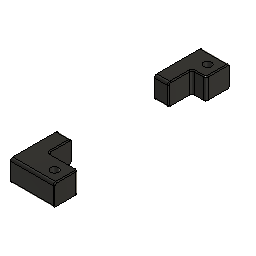
CableMount (Autodesk Fusion 360 design; units mm, degrees)
Autodesk Fusion 360 part; units mm, degrees
sketch "Sketch1" plane through (19.0523, 0, 0) normal (1, 0, 0) x (0, 1, 0)
  line L0 (120.65, 8.4918) -> (120.65, 16.9761)
  arc A0 (120.2964, 17.1226) -> (120.65, 16.9761) centre (120.65, 17.4761) ccw
  line L1 (120.2964, 17.1226) -> (118.5155, 18.9036)
  arc A1 (118.5155, 18.9036) -> (118.1619, 19.05) centre (118.1619, 18.55) ccw
  line L2 (118.1619, 19.05) -> (59.6381, 19.05)
  arc A2 (59.6381, 19.05) -> (59.2845, 18.9036) centre (59.6381, 18.55) ccw
  line L3 (59.2845, 18.9036) -> (57.5036, 17.1226)
  arc A3 (56.7964, 17.1226) -> (57.5036, 17.1226) centre (57.15, 17.4761) ccw
  line L4 (56.7964, 17.1226) -> (55.0155, 18.9036)
  arc A4 (55.0155, 18.9036) -> (54.6619, 19.05) centre (54.6619, 18.55) ccw
  line L5 (54.6619, 19.05) -> (-3.8619, 19.05)
  arc A5 (-3.8619, 19.05) -> (-4.2155, 18.9036) centre (-3.8619, 18.55) ccw
  line L6 (-4.2155, 18.9036) -> (-6.2036, 16.9155)
  arc A6 (-6.2036, 16.9155) -> (-6.35, 16.5619) centre (-5.85, 16.5619) ccw
  line L7 (-6.35, 16.5619) -> (-6.35, 7.4676)
  line L8 (-6.35, 7.4676) -> (56.1258, 7.4676)
  line L9 (56.1258, 7.4676) -> (57.15, 8.4918)
  line L10 (57.15, 8.4918) -> (58.1742, 7.4676)
  line L11 (58.1742, 7.4676) -> (119.6258, 7.4676)
  line L12 (119.6258, 7.4676) -> (120.65, 8.4918)
  line L13 (2.3114, 14.5034) -> (2.3114, 10.8966)
  arc A7 (1.8034, 10.3886) -> (2.3114, 10.8966) centre (1.8034, 10.8966) ccw
  line L14 (1.8034, 10.3886) -> (-1.8034, 10.3886)
  arc A8 (-2.3114, 10.8966) -> (-1.8034, 10.3886) centre (-1.8034, 10.8966) ccw
  line L15 (-2.3114, 10.8966) -> (-2.3114, 14.5034)
  arc A9 (-1.8034, 15.0114) -> (-2.3114, 14.5034) centre (-1.8034, 14.5034) ccw
  line L16 (-1.8034, 15.0114) -> (1.8034, 15.0114)
  arc A10 (2.3114, 14.5034) -> (1.8034, 15.0114) centre (1.8034, 14.5034) ccw
  line L17 (116.6114, 14.5034) -> (116.6114, 10.8966)
  arc A11 (116.1034, 10.3886) -> (116.6114, 10.8966) centre (116.1034, 10.8966) ccw
  line L18 (116.1034, 10.3886) -> (112.4966, 10.3886)
  arc A12 (111.9886, 10.8966) -> (112.4966, 10.3886) centre (112.4966, 10.8966) ccw
  line L19 (111.9886, 10.8966) -> (111.9886, 14.5034)
  arc A13 (112.4966, 15.0114) -> (111.9886, 14.5034) centre (112.4966, 14.5034) ccw
  line L20 (112.4966, 15.0114) -> (116.1034, 15.0114)
  arc A14 (116.6114, 14.5034) -> (116.1034, 15.0114) centre (116.1034, 14.5034) ccw
  line L21 (103.9114, 14.5034) -> (103.9114, 10.8966)
  arc A15 (103.4034, 10.3886) -> (103.9114, 10.8966) centre (103.4034, 10.8966) ccw
  line L22 (103.4034, 10.3886) -> (99.7966, 10.3886)
  arc A16 (99.2886, 10.8966) -> (99.7966, 10.3886) centre (99.7966, 10.8966) ccw
  line L23 (99.2886, 10.8966) -> (99.2886, 14.5034)
  arc A17 (99.7966, 15.0114) -> (99.2886, 14.5034) centre (99.7966, 14.5034) ccw
  line L24 (99.7966, 15.0114) -> (103.4034, 15.0114)
  arc A18 (103.9114, 14.5034) -> (103.4034, 15.0114) centre (103.4034, 14.5034) ccw
  line L25 (91.2114, 14.5034) -> (91.2114, 10.8966)
  arc A19 (90.7034, 10.3886) -> (91.2114, 10.8966) centre (90.7034, 10.8966) ccw
  line L26 (90.7034, 10.3886) -> (87.0966, 10.3886)
  arc A20 (86.5886, 10.8966) -> (87.0966, 10.3886) centre (87.0966, 10.8966) ccw
  line L27 (86.5886, 10.8966) -> (86.5886, 14.5034)
  arc A21 (87.0966, 15.0114) -> (86.5886, 14.5034) centre (87.0966, 14.5034) ccw
  line L28 (87.0966, 15.0114) -> (90.7034, 15.0114)
  arc A22 (91.2114, 14.5034) -> (90.7034, 15.0114) centre (90.7034, 14.5034) ccw
  line L29 (78.5114, 14.5034) -> (78.5114, 10.8966)
  arc A23 (78.0034, 10.3886) -> (78.5114, 10.8966) centre (78.0034, 10.8966) ccw
  line L30 (78.0034, 10.3886) -> (74.3966, 10.3886)
  arc A24 (73.8886, 10.8966) -> (74.3966, 10.3886) centre (74.3966, 10.8966) ccw
  line L31 (73.8886, 10.8966) -> (73.8886, 14.5034)
  arc A25 (74.3966, 15.0114) -> (73.8886, 14.5034) centre (74.3966, 14.5034) ccw
  line L32 (74.3966, 15.0114) -> (78.0034, 15.0114)
  arc A26 (78.5114, 14.5034) -> (78.0034, 15.0114) centre (78.0034, 14.5034) ccw
  line L33 (65.8114, 14.5034) -> (65.8114, 10.8966)
  arc A27 (65.3034, 10.3886) -> (65.8114, 10.8966) centre (65.3034, 10.8966) ccw
  line L34 (65.3034, 10.3886) -> (61.6966, 10.3886)
  arc A28 (61.1886, 10.8966) -> (61.6966, 10.3886) centre (61.6966, 10.8966) ccw
  line L35 (61.1886, 10.8966) -> (61.1886, 14.5034)
  arc A29 (61.6966, 15.0114) -> (61.1886, 14.5034) centre (61.6966, 14.5034) ccw
  line L36 (61.6966, 15.0114) -> (65.3034, 15.0114)
  arc A30 (65.8114, 14.5034) -> (65.3034, 15.0114) centre (65.3034, 14.5034) ccw
  line L37 (53.1114, 14.5034) -> (53.1114, 10.8966)
  arc A31 (52.6034, 10.3886) -> (53.1114, 10.8966) centre (52.6034, 10.8966) ccw
  line L38 (52.6034, 10.3886) -> (48.9966, 10.3886)
  arc A32 (48.4886, 10.8966) -> (48.9966, 10.3886) centre (48.9966, 10.8966) ccw
  line L39 (48.4886, 10.8966) -> (48.4886, 14.5034)
  arc A33 (48.9966, 15.0114) -> (48.4886, 14.5034) centre (48.9966, 14.5034) ccw
  line L40 (48.9966, 15.0114) -> (52.6034, 15.0114)
  arc A34 (53.1114, 14.5034) -> (52.6034, 15.0114) centre (52.6034, 14.5034) ccw
  line L41 (40.4114, 14.5034) -> (40.4114, 10.8966)
  arc A35 (39.9034, 10.3886) -> (40.4114, 10.8966) centre (39.9034, 10.8966) ccw
  line L42 (39.9034, 10.3886) -> (36.2966, 10.3886)
  arc A36 (35.7886, 10.8966) -> (36.2966, 10.3886) centre (36.2966, 10.8966) ccw
  line L43 (35.7886, 10.8966) -> (35.7886, 14.5034)
  arc A37 (36.2966, 15.0114) -> (35.7886, 14.5034) centre (36.2966, 14.5034) ccw
  line L44 (36.2966, 15.0114) -> (39.9034, 15.0114)
  arc A38 (40.4114, 14.5034) -> (39.9034, 15.0114) centre (39.9034, 14.5034) ccw
  line L45 (27.7114, 14.5034) -> (27.7114, 10.8966)
  arc A39 (27.2034, 10.3886) -> (27.7114, 10.8966) centre (27.2034, 10.8966) ccw
  line L46 (27.2034, 10.3886) -> (23.5966, 10.3886)
  arc A40 (23.0886, 10.8966) -> (23.5966, 10.3886) centre (23.5966, 10.8966) ccw
  line L47 (23.0886, 10.8966) -> (23.0886, 14.5034)
  arc A41 (23.5966, 15.0114) -> (23.0886, 14.5034) centre (23.5966, 14.5034) ccw
  line L48 (23.5966, 15.0114) -> (27.2034, 15.0114)
  arc A42 (27.7114, 14.5034) -> (27.2034, 15.0114) centre (27.2034, 14.5034) ccw
  line L49 (15.0114, 14.5034) -> (15.0114, 10.8966)
  arc A43 (14.5034, 10.3886) -> (15.0114, 10.8966) centre (14.5034, 10.8966) ccw
  line L50 (14.5034, 10.3886) -> (10.8966, 10.3886)
  arc A44 (10.3886, 10.8966) -> (10.8966, 10.3886) centre (10.8966, 10.8966) ccw
  line L51 (10.3886, 10.8966) -> (10.3886, 14.5034)
  arc A45 (10.8966, 15.0114) -> (10.3886, 14.5034) centre (10.8966, 14.5034) ccw
  line L52 (10.8966, 15.0114) -> (14.5034, 15.0114)
  arc A46 (15.0114, 14.5034) -> (14.5034, 15.0114) centre (14.5034, 14.5034) ccw
  line L53 (117.5722, 19.05) -> (119.38, 19.05)
  line L54 (120.65, 14.5095) -> (120.65, 17.78)
  line L55 (120.65, 14.5095) -> (120.65, 8.7341)
  line L56 (119.38, 7.4641) -> (96.52, 7.4641)
  line L57 (95.25, 8.7341) -> (95.25, 17.78)
  line L58 (96.52, 19.05) -> (117.5722, 19.05)
  arc A47 (120.65, 17.78) -> (119.38, 19.05) centre (119.38, 17.78) ccw
  arc A48 (119.38, 7.4641) -> (120.65, 8.7341) centre (119.38, 8.7341) ccw
  arc A49 (96.52, 19.05) -> (95.25, 17.78) centre (96.52, 17.78) ccw
  arc A50 (95.25, 8.7341) -> (96.52, 7.4641) centre (96.52, 8.7341) ccw
  point P0 (120.65, 7.4641)
  point P1 (95.25, 7.4641)
  dimension "d21" = 25.4
  dimension "d22" = 1.27
  constraint coincident L2 L53.start
  constraint coincident L0 L54.start
  constraint perpendicular L53 L54
  constraint perpendicular L11 L55
  constraint perpendicular L55 L56
  constraint perpendicular L2 L57
  constraint tangent L54 A47
  constraint tangent L53 A47
  constraint coincident P0 L55
  constraint coincident P0 L56
  constraint tangent L55 A48
  constraint tangent L56 A48
  constraint equal A47 A48
  constraint tangent L57 A49
  constraint tangent L58 A49
  constraint equal A47 A49
  constraint coincident P1 L56
  constraint coincident P1 L57
  constraint tangent L56 A50
  constraint tangent L57 A50
  constraint equal A47 A50
  measures "d21" distance of P0 P1
  measures "d22" radius of A47
extrude "Extrude1" add sketch "Sketch1" along normal blind 14.605 contours L0 A0 L1 A1 L2 L11 L12 L53 L54 L55 L57 L58 A48 A49 A50 | L12 A48 | A0 L1 A1 L53 L54 A47 | L17 A11 L18 A12 L19 A13 L20 A14 | L21 A15 L22 A16 L23 A17 L24 A18 makes body 1
sketch "Sketch2" plane through (0, 0, 7.4676) normal (0, 0, -1) x (1, 0, 0)
  line L0 (19.0523, -96.426) -> (19.0523, -119.474)
  line L1 (19.0523, -119.474) -> (33.6573, -119.474)
  line L2 (33.6573, -119.474) -> (33.6573, -96.426)
  line L3 (33.6573, -96.426) -> (19.0523, -96.426)
  line L4 (26.3548, -96.426) -> (26.3548, -107.856)
  line L5 (26.3548, -107.856) -> (33.6573, -107.856)
  line L6 (26.3548, -96.426) -> (26.3548, -95.1792)
  line L7 (26.3548, -95.1792) -> (33.6573, -95.1792)
  line L8 (33.6573, -95.1792) -> (33.6573, -107.856)
  dimension "d25" = 11.43
  dimension "d26" = 90
  constraint vertical L4
  constraint midpoint L3 L4.start
  constraint coincident L2 L5.end
  constraint perpendicular L3 L6
  constraint perpendicular L6 L7
  constraint perpendicular L5 L8
  measures "d25" distance of L4.start L4.end
  measures "d26" angle of L4 L5
extrude "Extrude2" cut sketch "Sketch2" against normal blind 29.6672 contours L3 L6 L7 L8 | L2 L3 L4 L5 L8 bodies 1
fillet "Fillet1" radius 1.27 2 edges at (26.3548, 107.856, 13.2588) (33.6573, 107.856, 13.2588) on bodies 1
fillet "Fillet2" radius 0.508 17 edges at (33.6573, 114.3, 7.4676) (33.2853, 108.228, 7.4676) (30.0061, 107.856, 7.4676) (26.7268, 107.4841, 7.4676) (26.3548, 101.506, 7.4676) (26.3548, 95.5893, 7.87) (26.3548, 95.25, 13.2571) (26.3548, 95.622, 18.678) (26.3548, 101.553, 19.05) (26.7268, 107.4841, 19.05) (30.0061, 107.856, 19.05) (33.2853, 108.228, 19.05) (33.6573, 114.253, 19.05) (33.6573, 120.278, 18.678) (33.6573, 120.65, 16.1448) (33.6573, 120.65, 11.6218) (33.6573, 120.3107, 7.87) on bodies 1
sketch "Sketch3" plane through (0, 0, 7.4676) normal (0, 0, -1) x (1, 0, 0)
  line L0 (33.1493, -119.474) -> (33.1493, -109.126)
  arc A0 (33.1493, -109.126) -> (32.3873, -108.364) centre (32.3873, -109.126) ccw
  line L1 (32.3873, -108.364) -> (27.6248, -108.364)
  arc A1 (25.8468, -106.586) -> (27.6248, -108.364) centre (27.6248, -106.586) ccw
  line L2 (25.8468, -106.586) -> (25.8468, -96.426)
  line L3 (25.8468, -96.426) -> (19.0523, -96.426)
  line L4 (19.0523, -96.426) -> (19.0523, -119.474)
  line L5 (19.0523, -119.474) -> (33.1493, -119.474)
  line L6 (30.2287, -114.3) -> (26.0385, -114.3)
  circle A2 centre (28.1336, -114.3) radius 2.0955
  dimension "d33" = 4.191
  constraint horizontal L6
  constraint midpoint L6 A2.centre
  measures "d33" diameter of A2
extrude "Extrude3" cut sketch "Sketch3" against normal blind 13.1318 contours L6 A2 | L6 A2 bodies 1
hole "Hole1" at (19.0523, 101.6, 12.7) direction (1, 0, 0) diameter 3.429 depth 6.35 tip angle 180 bodies 1
thread "Thread1" "ANSI Unified Screw Threads 0.164(#8) 8-32 UNC 8-32 UNC 2B" major diameter 4.1656 minor diameter 3.4163 pitch 0.7937 angle 60 modelled right hand crest width 0.2341 on face at (21.169, 101.738, 14.4089) crest through (19.2508, 99.8918, 12.7) on bodies 1
hole "Hole2" at (19.0523, 114.3, 12.7) direction (1, 0, 0) diameter 3.429 depth 6.35 tip angle 180 bodies 1
thread "Thread2" "ANSI Unified Screw Threads 0.164(#8) 8-32 UNC 8-32 UNC 2B" major diameter 4.1656 minor diameter 3.4163 pitch 0.7937 angle 60 modelled right hand crest width 0.2341 on face at (21.169, 115.194, 11.237) crest through (19.2508, 112.5918, 12.7) on bodies 1
sketch "Sketch4" plane through (19.0523, 0, 0) normal (1, 0, 0) x (0, 1, 0)
  line L0 (120.65, 8.4918) -> (120.65, 16.9761)
  arc A0 (120.2964, 17.1226) -> (120.65, 16.9761) centre (120.65, 17.4761) ccw
  line L1 (120.2964, 17.1226) -> (118.5155, 18.9036)
  arc A1 (118.5155, 18.9036) -> (118.1619, 19.05) centre (118.1619, 18.55) ccw
  line L2 (118.1619, 19.05) -> (59.6381, 19.05)
  arc A2 (59.6381, 19.05) -> (59.2845, 18.9036) centre (59.6381, 18.55) ccw
  line L3 (59.2845, 18.9036) -> (57.5036, 17.1226)
  arc A3 (56.7964, 17.1226) -> (57.5036, 17.1226) centre (57.15, 17.4761) ccw
  line L4 (56.7964, 17.1226) -> (55.0155, 18.9036)
  arc A4 (55.0155, 18.9036) -> (54.6619, 19.05) centre (54.6619, 18.55) ccw
  line L5 (54.6619, 19.05) -> (-3.8619, 19.05)
  arc A5 (-3.8619, 19.05) -> (-4.2155, 18.9036) centre (-3.8619, 18.55) ccw
  line L6 (-4.2155, 18.9036) -> (-6.2036, 16.9155)
  arc A6 (-6.2036, 16.9155) -> (-6.35, 16.5619) centre (-5.85, 16.5619) ccw
  line L7 (-6.35, 16.5619) -> (-6.35, 7.4676)
  line L8 (-6.35, 7.4676) -> (56.1258, 7.4676)
  line L9 (56.1258, 7.4676) -> (57.15, 8.4918)
  line L10 (57.15, 8.4918) -> (58.1742, 7.4676)
  line L11 (58.1742, 7.4676) -> (119.6258, 7.4676)
  line L12 (119.6258, 7.4676) -> (120.65, 8.4918)
  line L13 (2.3114, 14.5034) -> (2.3114, 10.8966)
  arc A7 (1.8034, 10.3886) -> (2.3114, 10.8966) centre (1.8034, 10.8966) ccw
  line L14 (1.8034, 10.3886) -> (-1.8034, 10.3886)
  arc A8 (-2.3114, 10.8966) -> (-1.8034, 10.3886) centre (-1.8034, 10.8966) ccw
  line L15 (-2.3114, 10.8966) -> (-2.3114, 14.5034)
  arc A9 (-1.8034, 15.0114) -> (-2.3114, 14.5034) centre (-1.8034, 14.5034) ccw
  line L16 (-1.8034, 15.0114) -> (1.8034, 15.0114)
  arc A10 (2.3114, 14.5034) -> (1.8034, 15.0114) centre (1.8034, 14.5034) ccw
  line L17 (116.6114, 14.5034) -> (116.6114, 10.8966)
  arc A11 (116.1034, 10.3886) -> (116.6114, 10.8966) centre (116.1034, 10.8966) ccw
  line L18 (116.1034, 10.3886) -> (112.4966, 10.3886)
  arc A12 (111.9886, 10.8966) -> (112.4966, 10.3886) centre (112.4966, 10.8966) ccw
  line L19 (111.9886, 10.8966) -> (111.9886, 14.5034)
  arc A13 (112.4966, 15.0114) -> (111.9886, 14.5034) centre (112.4966, 14.5034) ccw
  line L20 (112.4966, 15.0114) -> (116.1034, 15.0114)
  arc A14 (116.6114, 14.5034) -> (116.1034, 15.0114) centre (116.1034, 14.5034) ccw
  line L21 (103.9114, 14.5034) -> (103.9114, 10.8966)
  arc A15 (103.4034, 10.3886) -> (103.9114, 10.8966) centre (103.4034, 10.8966) ccw
  line L22 (103.4034, 10.3886) -> (99.7966, 10.3886)
  arc A16 (99.2886, 10.8966) -> (99.7966, 10.3886) centre (99.7966, 10.8966) ccw
  line L23 (99.2886, 10.8966) -> (99.2886, 14.5034)
  arc A17 (99.7966, 15.0114) -> (99.2886, 14.5034) centre (99.7966, 14.5034) ccw
  line L24 (99.7966, 15.0114) -> (103.4034, 15.0114)
  arc A18 (103.9114, 14.5034) -> (103.4034, 15.0114) centre (103.4034, 14.5034) ccw
  line L25 (91.2114, 14.5034) -> (91.2114, 10.8966)
  arc A19 (90.7034, 10.3886) -> (91.2114, 10.8966) centre (90.7034, 10.8966) ccw
  line L26 (90.7034, 10.3886) -> (87.0966, 10.3886)
  arc A20 (86.5886, 10.8966) -> (87.0966, 10.3886) centre (87.0966, 10.8966) ccw
  line L27 (86.5886, 10.8966) -> (86.5886, 14.5034)
  arc A21 (87.0966, 15.0114) -> (86.5886, 14.5034) centre (87.0966, 14.5034) ccw
  line L28 (87.0966, 15.0114) -> (90.7034, 15.0114)
  arc A22 (91.2114, 14.5034) -> (90.7034, 15.0114) centre (90.7034, 14.5034) ccw
  line L29 (78.5114, 14.5034) -> (78.5114, 10.8966)
  arc A23 (78.0034, 10.3886) -> (78.5114, 10.8966) centre (78.0034, 10.8966) ccw
  line L30 (78.0034, 10.3886) -> (74.3966, 10.3886)
  arc A24 (73.8886, 10.8966) -> (74.3966, 10.3886) centre (74.3966, 10.8966) ccw
  line L31 (73.8886, 10.8966) -> (73.8886, 14.5034)
  arc A25 (74.3966, 15.0114) -> (73.8886, 14.5034) centre (74.3966, 14.5034) ccw
  line L32 (74.3966, 15.0114) -> (78.0034, 15.0114)
  arc A26 (78.5114, 14.5034) -> (78.0034, 15.0114) centre (78.0034, 14.5034) ccw
  line L33 (65.8114, 14.5034) -> (65.8114, 10.8966)
  arc A27 (65.3034, 10.3886) -> (65.8114, 10.8966) centre (65.3034, 10.8966) ccw
  line L34 (65.3034, 10.3886) -> (61.6966, 10.3886)
  arc A28 (61.1886, 10.8966) -> (61.6966, 10.3886) centre (61.6966, 10.8966) ccw
  line L35 (61.1886, 10.8966) -> (61.1886, 14.5034)
  arc A29 (61.6966, 15.0114) -> (61.1886, 14.5034) centre (61.6966, 14.5034) ccw
  line L36 (61.6966, 15.0114) -> (65.3034, 15.0114)
  arc A30 (65.8114, 14.5034) -> (65.3034, 15.0114) centre (65.3034, 14.5034) ccw
  line L37 (53.1114, 14.5034) -> (53.1114, 10.8966)
  arc A31 (52.6034, 10.3886) -> (53.1114, 10.8966) centre (52.6034, 10.8966) ccw
  line L38 (52.6034, 10.3886) -> (48.9966, 10.3886)
  arc A32 (48.4886, 10.8966) -> (48.9966, 10.3886) centre (48.9966, 10.8966) ccw
  line L39 (48.4886, 10.8966) -> (48.4886, 14.5034)
  arc A33 (48.9966, 15.0114) -> (48.4886, 14.5034) centre (48.9966, 14.5034) ccw
  line L40 (48.9966, 15.0114) -> (52.6034, 15.0114)
  arc A34 (53.1114, 14.5034) -> (52.6034, 15.0114) centre (52.6034, 14.5034) ccw
  line L41 (40.4114, 14.5034) -> (40.4114, 10.8966)
  arc A35 (39.9034, 10.3886) -> (40.4114, 10.8966) centre (39.9034, 10.8966) ccw
  line L42 (39.9034, 10.3886) -> (36.2966, 10.3886)
  arc A36 (35.7886, 10.8966) -> (36.2966, 10.3886) centre (36.2966, 10.8966) ccw
  line L43 (35.7886, 10.8966) -> (35.7886, 14.5034)
  arc A37 (36.2966, 15.0114) -> (35.7886, 14.5034) centre (36.2966, 14.5034) ccw
  line L44 (36.2966, 15.0114) -> (39.9034, 15.0114)
  arc A38 (40.4114, 14.5034) -> (39.9034, 15.0114) centre (39.9034, 14.5034) ccw
  line L45 (27.7114, 14.5034) -> (27.7114, 10.8966)
  arc A39 (27.2034, 10.3886) -> (27.7114, 10.8966) centre (27.2034, 10.8966) ccw
  line L46 (27.2034, 10.3886) -> (23.5966, 10.3886)
  arc A40 (23.0886, 10.8966) -> (23.5966, 10.3886) centre (23.5966, 10.8966) ccw
  line L47 (23.0886, 10.8966) -> (23.0886, 14.5034)
  arc A41 (23.5966, 15.0114) -> (23.0886, 14.5034) centre (23.5966, 14.5034) ccw
  line L48 (23.5966, 15.0114) -> (27.2034, 15.0114)
  arc A42 (27.7114, 14.5034) -> (27.2034, 15.0114) centre (27.2034, 14.5034) ccw
  line L49 (15.0114, 14.5034) -> (15.0114, 10.8966)
  arc A43 (14.5034, 10.3886) -> (15.0114, 10.8966) centre (14.5034, 10.8966) ccw
  line L50 (14.5034, 10.3886) -> (10.8966, 10.3886)
  arc A44 (10.3886, 10.8966) -> (10.8966, 10.3886) centre (10.8966, 10.8966) ccw
  line L51 (10.3886, 10.8966) -> (10.3886, 14.5034)
  arc A45 (10.8966, 15.0114) -> (10.3886, 14.5034) centre (10.8966, 14.5034) ccw
  line L52 (10.8966, 15.0114) -> (14.5034, 15.0114)
  arc A46 (15.0114, 14.5034) -> (14.5034, 15.0114) centre (14.5034, 14.5034) ccw
  line L53 (-6.35, 12.0148) -> (-6.35, 19.05)
  line L54 (-5.08, 19.05) -> (17.78, 19.05)
  line L55 (19.05, 8.7376) -> (19.05, 17.78)
  line L56 (17.78, 7.4676) -> (-5.08, 7.4676)
  line L57 (-6.35, 8.7376) -> (-6.35, 17.78)
  arc A47 (-5.08, 19.05) -> (-6.35, 17.78) centre (-5.08, 17.78) ccw
  arc A48 (-6.35, 8.7376) -> (-5.08, 7.4676) centre (-5.08, 8.7376) ccw
  arc A49 (19.05, 17.78) -> (17.78, 19.05) centre (17.78, 17.78) ccw
  arc A50 (17.78, 7.4676) -> (19.05, 8.7376) centre (17.78, 8.7376) ccw
  point P0 (19.05, 19.05)
  dimension "d46" = 25.4
  dimension "d47" = 1.27
  constraint midpoint L7 L53.start
  constraint perpendicular L5 L53
  constraint perpendicular L53 L54
  constraint perpendicular L54 L55
  constraint coincident L53.end L54
  constraint coincident L53.end L57
  constraint tangent L54 A47
  constraint tangent L57 A47
  constraint tangent L56 A48
  constraint tangent L57 A48
  constraint equal A47 A48
  constraint coincident P0 L54
  constraint coincident P0 L55
  constraint tangent L54 A49
  constraint tangent L55 A49
  constraint equal A47 A49
  constraint tangent L55 A50
  constraint tangent L56 A50
  constraint equal A47 A50
  measures "d46" distance of L53.end P0
  measures "d47" radius of A47
extrude "Extrude4" add sketch "Sketch4" along normal blind 27.305 separate body contours L5 A5 L6 A6 L7 L8 L53 L54 L55 L56 L57 A48 A49 A50 | A5 L6 A6 L53 L54 L57 A47 | L13 A7 L14 A8 L15 A9 L16 A10 | L49 A43 L50 A44 L51 A45 L52 A46 makes body 2
sketch "Sketch5" plane through (0, 0, 7.4676) normal (0, 0, -1) x (1, 0, 0)
  line L0 (19.0523, 5.08) -> (19.0523, -17.78)
  line L1 (19.0523, -17.78) -> (46.3573, -17.78)
  line L2 (46.3573, -17.78) -> (46.3573, 5.08)
  line L3 (46.3573, 5.08) -> (19.0523, 5.08)
  line L4 (26.3242, -96.7096) -> (26.3242, -17.78)
  line L5 (26.3242, -17.78) -> (46.3573, -17.78)
  line L6 (46.3573, -6.35) -> (19.0523, -6.35)
  line L7 (19.0523, -17.78) -> (19.0523, -19.5515)
  line L8 (19.0523, -19.5515) -> (46.3573, -19.5515)
  line L9 (46.3573, -19.5515) -> (46.3573, -17.78)
  line L10 (46.3573, -20.824) -> (46.3573, -7.616)
  line L11 (46.3573, -7.616) -> (19.0523, -7.616)
  line L12 (19.0523, -7.616) -> (19.0523, -19.5515)
  line L13 (26.3242, -17.78) -> (26.3242, -7.616)
  line L14 (26.3242, -7.616) -> (26.3242, -6.35)
  line L15 (46.3573, -7.616) -> (42.1346, -7.616)
  line L16 (42.1346, -7.616) -> (42.1346, 6.5274)
  line L17 (42.1346, 6.5274) -> (46.3573, 6.5274)
  line L18 (46.3573, 6.5274) -> (46.3573, -7.616)
  dimension "d54" = 13.208
  dimension "d55" = 90
  dimension "d96" = 4.2227
  constraint coincident L1 L4.end
  constraint perpendicular L1 L4
  constraint coincident L1.end L2.start
  constraint midpoint L2 L6.start
  constraint midpoint L0 L6.end
  constraint perpendicular L1 L7
  constraint perpendicular L4 L8
  constraint perpendicular L5 L9
  constraint coincident L9 L10.start
  constraint perpendicular L8 L10
  constraint coincident L0 L11.end
  constraint coincident L11 L13.end
  constraint perpendicular L11 L13
  constraint coincident L6 L14.end
  constraint perpendicular L6 L14
  constraint coincident L11 L15.end
  constraint perpendicular L3 L16
  constraint perpendicular L16 L17
  constraint perpendicular L11 L18
  measures "d54" distance of L10.start L10.end
  measures "d55" angle of L10 L11
  measures "d96" distance of L10.end L15.end
extrude "Extrude6" cut sketch "Sketch5" against normal blind 36.957 contours L3 L16 L17 L18 | L2 L3 L6 L16 L18 | L6 L11 L14 L16 | L2 L6 L11 L15 L16 L18 | L1 L2 L5 L10 L11 L13 L15 | L1 L4 L5 L8 L9 L10 bodies 2
sketch "Sketch6" plane through (0, 0, 7.4676) normal (0, 0, -1) x (1, 0, 0)
  line L0 (42.1346, 5.08) -> (19.0523, 5.08)
  line L1 (19.0523, 5.08) -> (19.0523, -17.78)
  line L2 (19.0523, -17.78) -> (26.3242, -17.78)
  line L3 (36.0705, 0) -> (36.0701, 0)
  circle A0 centre (36.0703, 0) radius 2.0955
  line L4 (36.0705, 0) -> (45.8493, 0)
  line L5 (45.8493, 0) -> (36.0703, 0)
  line L6 (42.1346, -6.35) -> (42.1346, 5.08)
  line L7 (26.3242, -17.78) -> (26.3242, -6.35)
  line L8 (26.3242, -6.35) -> (42.1346, -6.35)
  dimension "d66" = 4.191
  dimension "d95" = 9.779
  constraint midpoint L3 A0.centre
  constraint coincident L4 A0.centre
  constraint coincident A0.centre L5.end
  measures "d66" diameter of A0
  measures "d95" distance of L4.end A0.centre
extrude "Extrude7" cut sketch "Sketch6" against normal blind 17.0942 contours A0 bodies 2
hole "Hole3" at (19.0523, 0, 12.7) direction (1, 0, 0) diameter 3.429 depth 9.525 tip angle 180 bodies 2
thread "Thread3" "ANSI Unified Screw Threads 0.164(#8) 8-32 UNC 8-32 UNC 2B" major diameter 4.1656 minor diameter 3.4163 pitch 0.7937 angle 60 modelled right hand crest width 0.2341 on face at (22.2273, 0.1707, 14.406) crest through (19.2508, -1.7082, 12.7) on bodies 2
hole "Hole4" at (19.0523, 12.7, 12.7) direction (1, 0, 0) diameter 3.429 depth 6.35 tip angle 180 bodies 2
thread "Thread4" "ANSI Unified Screw Threads 0.164(#8) 8-32 UNC 8-32 UNC 2B" major diameter 4.1656 minor diameter 3.4163 pitch 0.7937 angle 60 modelled right hand crest width 0.2341 on face at (21.169, 12.8707, 14.406) crest through (19.2508, 10.9918, 12.7) on bodies 2
move_body "Move1" bodies 1 to x (1, 0, 0) y (0, 1, 0) z (0, 0, 1) at (0, -25.4, 0)
fillet "Fillet7" radius 1.27 2 edges at (42.1346, 6.35, 13.2588) (26.3242, 6.35, 13.2588) on bodies 2
fillet "Fillet8" radius 0.508 16 edges at (42.1346, -6.35, 13.2588) (42.1346, -5.978, 18.678) (42.1346, 0, 19.05) (41.7626, 5.978, 19.05) (34.2294, 6.35, 19.05) (26.6962, 6.722, 19.05) (26.3242, 12.7, 19.05) (26.3242, 18.678, 18.678) (26.3242, 19.05, 13.2588) (26.3242, 18.678, 7.8396) (26.3242, 12.7, 7.4676) (26.6962, 6.722, 7.4676) (34.2294, 6.35, 7.4676) (41.7626, 5.978, 7.4676) (42.1346, 0, 7.4676) (42.1346, -5.978, 7.8396) on bodies 2
equation "d95 = 0.115 in + 0.1875 in + 0.0825 in"
equation "d96 = ( ( 0.0625 in + 0.1875 in + 0.0825 in ) / 2 in ) * 1 in"
named bodies: "CableMount1", "CableMount2"
